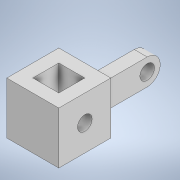
# Autodesk Inventor part: CAM03
Saved by Autodesk Inventor 2020.3 (Build 243373000, 373)
## iProperties
Created: 2021-05-24
Part Number: CAM03
Material: Generic
Document SubType Name: Modeling
Designer: patry
Density: 1 g/cm^3
Appearance: Default
Author: patry
Autodesk Inventor part; units mm, degrees
ref_plane "YZ Plane" through (0, 0, 0) normal (1, 0, 0) x (0, 1, 0)
ref_plane "XZ Plane" through (0, 0, 0) normal (0, 1, 0) x (-1, 0, 0)
ref_plane "XY Plane" through (0, 0, 0) normal (0, 0, 1) x (1, 0, 0)
sketch "Sketch1" plane through (0, 0, 0) normal (0, 1, 0) x (-1, 0, 0)
  line L0 (0, 0) -> (-10, 0)
  line L1 (-10, 0) -> (-10, 10)
  line L2 (-10, 10) -> (0, 10)
  line L3 (0, 10) -> (0, 0)
  line L4 (0, 0) -> (-2.5, 0)
  line L5 (-2.5, 0) -> (-2.5, 2.5)
  line L6 (-2.5, 2.5) -> (0, 2.5)
  line L7 (0, 2.5) -> (0, 0)
  line L8 (-2.5, 2.5) -> (-7.5, 2.5)
  line L9 (-7.5, 2.5) -> (-7.5, 7.5)
  line L10 (-7.5, 7.5) -> (-2.5, 7.5)
  line L11 (-2.5, 7.5) -> (-2.5, 2.5)
  dimension "d0" = 10
  dimension "d1" = 10
  dimension "d2" = 2.5
  dimension "d3" = 2.5
  dimension "d4" = 5
  dimension "d5" = 5
  constraints: 24 end point, 6 parallel, 3 horizontal, 3 perpendicular
  measures "d0" distance of L1.end L2.end
  measures "d1" distance of L0.end L1.end
  measures "d2" distance of L5.end L6.end
  measures "d3" distance of L4.end L5.end
  measures "d4" distance of L9.end L10.end
  measures "d5" distance of L8.end L9.end
extrude "Extrusion1" add sketch "Sketch1" along normal blind 10
sketch "Sketch2" plane through (10, 0, 10) normal (1, 0, 0) x (0, 0, -1)
  line L0 (10, 10) -> (0, 10) projected
  line L1 (0, 10) -> (5, 10)
  line L2 (5, 10) -> (5, 5)
  line L3 (5, 5) -> (0, 5)
  line L4 (0, 5) -> (0, 10)
  circle A0 centre (5, 5) radius 1.4
  point P0 (10, 0)
  dimension "d8" = 5
  dimension "d9" = 5
  dimension "d10" = 2.8
  constraints: 8 end point, 2 parallel, 1 centre point, 1 coincident, 1 horizontal, 1 perpendicular
  measures "d8" distance of L2.end L3.end
  measures "d9" distance of L1.end L2.end
  measures "d10" diameter of A0
extrude "Extrusion2" cut sketch "Sketch2" against normal through all contours A0 L3 L2 | L2 L3 A0
sketch "Sketch3" plane through (10, 0, 0) normal (0, 0, -1) x (-1, 0, 0)
  line L0 (0, 10) -> (10, 10) projected
  line L1 (10, 10) -> (7.5, 10)
  line L2 (7.5, 10) -> (7.5, 7.5)
  line L3 (7.5, 7.5) -> (10, 7.5)
  line L4 (10, 7.5) -> (10, 10)
  line L5 (7.5, 7.5) -> (2.5, 7.5)
  line L6 (2.5, 7.5) -> (2.5, 2.5)
  line L7 (2.5, 2.5) -> (7.5, 2.5)
  line L8 (7.5, 2.5) -> (7.5, 7.5)
  line L9 (2.5, 2.5) -> (5, 2.5)
  line L10 (5, 2.5) -> (5, 7.5)
  line L11 (5, 7.5) -> (2.5, 7.5)
  line L12 (2.5, 7.5) -> (2.5, 2.5)
  point P0 (10, 0)
  dimension "d13" = 2.5
  dimension "d14" = 2.5
  dimension "d15" = 5
  dimension "d16" = 5
  constraints: 24 end point, 6 parallel, 3 horizontal, 3 perpendicular, 1 midpoint
  measures "d13" distance of L3.end L2.end
  measures "d14" distance of L2.end L1.end
  measures "d15" distance of L7.end L6.end
  measures "d16" distance of L6.end L5.end
extrude "Extrusion3" add sketch "Sketch3" along normal blind 12 contours L10 L7 L6 L5
sketch "Sketch4" plane through (7.5, 2.5, 0) normal (1, 0, 0) x (0, 0, -1)
  line L0 (0, 5) -> (12, 5) projected
  line L1 (12, 5) -> (9.5, 5)
  line L2 (9.5, 5) -> (9.5, 2.5)
  line L3 (9.5, 2.5) -> (12, 2.5)
  line L4 (12, 2.5) -> (12, 5)
  circle A0 centre (9.5, 2.5) radius 1.4
  point P0 (0, -2.5)
  dimension "d19" = 2.5
  dimension "d20" = 2.5
  dimension "d21" = 2.8
  constraints: 8 end point, 2 parallel, 1 centre point, 1 coincident, 1 horizontal, 1 perpendicular
  measures "d19" distance of L3.end L2.end
  measures "d20" distance of L2.end L1.end
  measures "d21" diameter of A0
extrude "Extrusion4" cut sketch "Sketch4" against normal through all contours A0 L3 L2 | L2 L3 A0
fillet "Fillet1" radius 2.5 2 edges at (6.25, 7.5, -12) (6.25, 2.5, -12)
body "Solid1"
